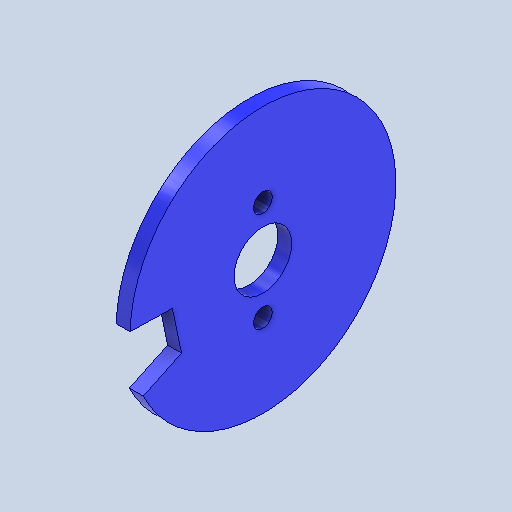
# Autodesk Inventor part: belt_liner_v2_3DP_P-4-F
Saved by Autodesk Inventor 2025.2 (Build 292293000, 293)
## iProperties
Created: 2025-01-13
Part Number: belt_liner_v2_3DP_P-4-F
Material: ABS プラスチック
Document SubType Name: Modeling
Designer: haruy
Density: 1.06 g/cm^3
Appearance: 青 - 壁塗料 - 光沢
Author: haruy
Autodesk Inventor part; units mm, degrees
ref_plane "YZ Plane" through (0, 0, 0) normal (1, 0, 0) x (0, 1, 0)
ref_plane "XZ Plane" through (0, 0, 0) normal (0, 1, 0) x (-1, 0, 0)
ref_plane "XY Plane" through (0, 0, 0) normal (0, 0, 1) x (1, 0, 0)
sketch "スケッチ1" plane through (0, 0, 0) normal (1, 0, 0) x (0, 1, 0)
  line L0 (-2.8814, 19.0389) -> (-6.1428, 25.9541)
  arc A0 (-6.1428, 25.9541) -> (5.1106, 28.346) centre (4.3283, 4.3588) ccw
  line L1 (5.1106, 28.346) -> (4.9438, 20.7022)
  line L2 (4.9438, 20.7022) -> (-2.8814, 19.0389)
  circle A1 centre (-4.6717, 4.3588) radius 1.7
  circle A2 centre (13.3283, 4.3588) radius 1.7
  circle A3 centre (4.3283, 4.3588) radius 5.2
  point P0 (0, 0)
  constraints: 6 end point, 4 centre point, 2 point on circle
extrude "押し出し1" add sketch "スケッチ1" along normal blind 2.5
